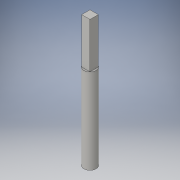
# Autodesk Inventor part: shaft_adapter_v2
Saved by Autodesk Inventor 2016 (Build 200138000, 138)
## iProperties
Created: 2015-12-10
Part Number: shaft_adapter_v2
Material: Generic
Document SubType Name: Modeling
Designer: jfranz
Density: 1 g/cm^3
Appearance: Default
Author: jfranz
Autodesk Inventor part; units mm, degrees
ref_plane "YZ Plane" through (0, 0, 0) normal (1, 0, 0) x (0, 1, 0)
ref_plane "XZ Plane" through (0, 0, 0) normal (0, 1, 0) x (-1, 0, 0)
ref_plane "XY Plane" through (0, 0, 0) normal (0, 0, 1) x (1, 0, 0)
sketch "Sketch1" plane through (0, 0, 0) normal (0, 1, 0) x (-1, 0, 0)
  circle A0 centre (0, 0) radius 2.032
  dimension "d0" = 4.064
  constraints: 1 centre point, 1 coincident
  measures "d0" diameter of A0
extrude "Extrusion1" add sketch "Sketch1" along normal blind 28.575
sketch "Sketch2" plane through (0, 28.575, 0) normal (0, 1, 0) x (1, 0, 0)
  line L0 (-1.397, -1.397) -> (1.397, -1.397)
  line L1 (1.397, -1.397) -> (1.397, 1.397)
  line L2 (1.397, 1.397) -> (-1.397, 1.397)
  line L3 (-1.397, 1.397) -> (-1.397, -1.397)
  point P0 (0, 0)
  point P1 (-1.397, 0)
  point P2 (0, -1.397)
  dimension "d3" = 2.794
  dimension "d4" = 2.794
  constraints: 8 end point, 2 midpoint, 2 parallel, 1 horizontal, 1 horizontal alignment, 1 perpendicular, 1 vertical alignment
  measures "d3" distance of L0.start L0.end
  measures "d4" distance of L2.end L0.start
extrude "Extrusion2" add sketch "Sketch2" along normal blind 15.24
sketch "Sketch3" plane through (0, 0, 0) normal (0, -1, 0) x (1, 0, 0)
  point P0 (0, 0)
  point P1 (0, 0)
  constraints: 1 coincident
hole "Hole1" at (0, 0, 0) direction (0, 1, 0) diameter 2.413 depth 26.67
equation "\"d4\" = d3"
body "Solid1"
